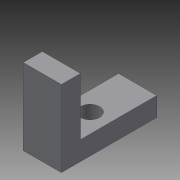
# Autodesk Inventor part: Угловой_крепеж
Saved by Autodesk Inventor 2014 (Build 180170000, 170)
## iProperties
Created: 2017-02-08
Part Number: Угловой_крепеж
Material: Типовые
Document SubType Name: Modeling
Designer: Nikopol
Density: 1 g/cm^3
Appearance: По умолчанию
Author: Nikopol
Autodesk Inventor part; units mm, degrees
ref_plane "YZ Plane" through (0, 0, 0) normal (1, 0, 0) x (0, 1, 0)
ref_plane "XZ Plane" through (0, 0, 0) normal (0, 1, 0) x (-1, 0, 0)
ref_plane "XY Plane" through (0, 0, 0) normal (0, 0, 1) x (1, 0, 0)
sketch "Эскиз1" plane through (0, 0, 0) normal (0, 0, 1) x (1, 0, 0)
  line L0 (-3, 7.5) -> (3, 7.5)
  line L1 (3, 7.5) -> (3, -7.5)
  line L2 (3, -7.5) -> (-3, -7.5)
  line L3 (-3, -7.5) -> (-3, 7.5)
  point P0 (0, 0)
  point P1 (3, 0)
  point P2 (0, 7.5)
  dimension "d0" = 6
  dimension "d1" = 15
  constraints: 8 end point, 2 midpoint, 2 parallel, 1 horizontal, 1 horizontal alignment, 1 perpendicular, 1 vertical alignment
  measures "d0" distance of L1.end L2.end
  measures "d1" distance of L0.end L1.end
extrude "Выдавливание1" add sketch "Эскиз1" along normal blind 3
sketch "Эскиз2" plane through (0, 0, 3) normal (0, 0, 1) x (1, 0, 0)
  line L0 (3, 7.5) -> (-3, 7.5) projected
  point P0 (0, 0)
  point P1 (0, 0)
  dimension "d4" = 7.5
  measures "d4" distance from line of L0 point (0, 0)
hole "Отверстие1" at (0, 0, 3) direction (0, 0, -1) diameter 3 end through all
sketch "Эскиз3" plane through (0, 0, 3) normal (0, 0, 1) x (1, 0, 0)
  line L0 (3, -7.5) -> (3, 7.5) projected
  line L1 (-3, -7.5) -> (3, -7.5)
  line L2 (3, -7.5) -> (3, -4.5)
  line L3 (3, -4.5) -> (-3, -4.5)
  line L4 (-3, -4.5) -> (-3, -7.5)
  dimension "d12" = 3
  constraints: 8 end point, 2 parallel, 1 horizontal, 1 perpendicular, 1 point on line
  measures "d12" distance of L2.end L1.end
extrude "Выдавливание2" add sketch "Эскиз3" along normal blind 9
